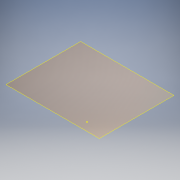
# Autodesk Inventor part: headers
Saved by Autodesk Inventor 2016 (Build 200138000, 138)
## iProperties
Created: 2016-04-08
Part Number: headers
Material: Generic
Document SubType Name: Modeling
Designer: Paschalis
Density: 1 g/cm^3
Appearance: Gold
Author: Paschalis
Autodesk Inventor part; units mm, degrees
ref_plane "YZ Plane" through (0, 0, 0) normal (1, 0, 0) x (0, 1, 0)
ref_plane "XZ Plane" through (0, 0, 0) normal (0, 1, 0) x (-1, 0, 0)
ref_plane "XY Plane" through (0, 0, 0) normal (0, 0, 1) x (1, 0, 0)
ref_plane "Work Plane1" through (-30.9119, 34.3331, -1) normal (0, 0, 1) x (-1, 0, 0)
sketch "Sketch1" plane through (-30.9119, 34.3331, -1) normal (0, 0, 1) x (-1, 0, 0)
  circle A0 centre (43.25, -35) radius 1.8 projected
  circle A1 centre (-43.25, 35) radius 1.8 projected
  circle A2 centre (-43.25, -35) radius 1.8 projected
  circle A3 centre (30.74, 18.1) radius 0.8 projected
  circle A4 centre (23.98, 18.1) radius 0.8 projected
  circle A5 centre (40.4, 18.1) radius 0.8 projected
  circle A6 centre (47.16, 18.1) radius 0.8 projected
  circle A7 centre (33.82, 25.76) radius 0.75 projected
  circle A8 centre (33.82, 35.92) radius 0.75 projected
  circle A9 centre (43.98, 25.76) radius 0.75 projected
  circle A10 centre (43.98, 35.92) radius 0.75 projected
  circle A11 centre (12.23, 25.76) radius 0.75 projected
  circle A12 centre (12.23, 35.92) radius 0.75 projected
  circle A13 centre (22.39, 25.76) radius 0.75 projected
  circle A14 centre (22.39, 35.92) radius 0.75 projected
  circle A15 centre (-36.03, -34.92) radius 0.55 projected
  circle A16 centre (-38.57, -34.92) radius 0.55 projected
  circle A17 centre (-7.7725, -36.5075) radius 0.55 projected
  circle A18 centre (40.805, -30.475) radius 0.55 projected
  circle A19 centre (-11.9, -36.19) radius 0.55 projected
  circle A20 centre (-14.44, -36.19) radius 0.55 projected
  circle A21 centre (-16.98, -36.19) radius 0.55 projected
  circle A22 centre (-11.9, -38.73) radius 0.55 projected
  circle A23 centre (-14.44, -38.73) radius 0.55 projected
  circle A24 centre (-16.98, -38.73) radius 0.55 projected
  circle A25 centre (-8.8, -11.34) radius 0.51 projected
  circle A26 centre (-11.34, -11.34) radius 0.51 projected
  circle A27 centre (-45.55, -7.62) radius 0.51 projected
  circle A28 centre (-43.01, -7.62) radius 0.51 projected
  circle A29 centre (-45.55, -10.15) radius 0.51 projected
  circle A30 centre (-43.01, -10.15) radius 0.51 projected
  circle A31 centre (-45.55, -12.7) radius 0.51 projected
  circle A32 centre (-43.01, -12.7) radius 0.51 projected
  circle A33 centre (-45.55, -15.23) radius 0.51 projected
  circle A34 centre (-43.01, -15.23) radius 0.51 projected
  circle A35 centre (-1.1, 23.5) radius 0.51 projected
  circle A36 centre (1.44, 23.5) radius 0.51 projected
  circle A37 centre (3.98, 23.5) radius 0.51 projected
  circle A38 centre (-12.22, 23.5) radius 0.51 projected
  circle A39 centre (-9.68, 23.5) radius 0.51 projected
  circle A40 centre (-7.14, 23.5) radius 0.51 projected
  circle A41 centre (3.98, 33.66) radius 0.51 projected
  circle A42 centre (1.44, 33.66) radius 0.51 projected
  circle A43 centre (-1.1, 33.66) radius 0.51 projected
  circle A44 centre (-7.14, 33.66) radius 0.51 projected
  circle A45 centre (-9.68, 33.66) radius 0.51 projected
  circle A46 centre (-12.22, 33.66) radius 0.51 projected
  circle A47 centre (-34.76, 33.03) radius 0.51 projected
  circle A48 centre (-34.76, 35.56) radius 0.51 projected
  circle A49 centre (-32.22, 33.03) radius 0.51 projected
  circle A50 centre (-32.22, 35.56) radius 0.51 projected
  circle A51 centre (-29.68, 33.03) radius 0.51 projected
  circle A52 centre (-29.68, 35.56) radius 0.51 projected
  circle A53 centre (-27.14, 33.03) radius 0.51 projected
  circle A54 centre (-27.14, 35.56) radius 0.51 projected
  circle A55 centre (-40.47, -20.31) radius 0.51 projected
  circle A56 centre (-40.47, -22.86) radius 0.51 projected
  circle A57 centre (-43.01, -20.31) radius 0.51 projected
  circle A58 centre (-43.01, -22.86) radius 0.51 projected
  circle A59 centre (-45.55, -20.31) radius 0.51 projected
  circle A60 centre (-45.55, -22.86) radius 0.51 projected
  circle A61 centre (33.82, -10.15) radius 0.51 projected
  circle A62 centre (33.82, -12.7) radius 0.51 projected
  circle A63 centre (33.82, -15.23) radius 0.51 projected
  circle A64 centre (33.82, -17.77) radius 0.51 projected
  circle A65 centre (10.33, -1.9) radius 0.51 projected
  circle A66 centre (10.33, 0.64) radius 0.51 projected
  circle A67 centre (-25.36, -29.21) radius 0.405 projected
  circle A68 centre (-30.19, -29.21) radius 0.405 projected
  circle A69 centre (19.98, -20.95) radius 0.405 projected
  circle A70 centre (24.8, -20.95) radius 0.405 projected
  circle A71 centre (40.4875, 22.5475) radius 0.3 projected
  circle A72 centre (43.98, 16.8325) radius 0.3 projected
  circle A73 centre (43.98, 19.69) radius 0.3 projected
  circle A74 centre (43.98, 22.5475) radius 0.3 projected
  circle A75 centre (47.155, 26.675) radius 0.3 projected
  circle A76 centre (47.155, 31.12) radius 0.3 projected
  circle A77 centre (43.345, 31.12) radius 0.3 projected
  circle A78 centre (47.155, 35.565) radius 0.3 projected
  circle A79 centre (47.79, 22.5475) radius 0.3 projected
  circle A80 centre (30.3275, 29.215) radius 0.3 projected
  circle A81 centre (1.435, 38.4225) radius 0.3 projected
  circle A82 centre (34.1375, 33.025) radius 0.3 projected
  circle A83 centre (21.755, 33.025) radius 0.3 projected
  circle A84 centre (25.565, 29.215) radius 0.3 projected
  circle A85 centre (21.755, 29.215) radius 0.3 projected
  circle A86 centre (25.565, 33.025) radius 0.3 projected
  circle A87 centre (30.3275, 33.025) radius 0.3 projected
  circle A88 centre (34.1375, 29.215) radius 0.3 projected
  circle A89 centre (28.105, 36.5175) radius 0.3 projected
  circle A90 centre (28.105, 25.0875) radius 0.3 projected
  circle A91 centre (-20.79, -12.3775) radius 0.3 projected
  circle A92 centre (-24.9175, -10.4725) radius 0.3 projected
  circle A93 centre (-24.6, -8.25) radius 0.3 projected
  circle A94 centre (-2.375, -13.965) radius 0.3 projected
  circle A95 centre (-30.315, -13.965) radius 0.3 projected
  circle A96 centre (-19.52, -11.425) radius 0.3 projected
  circle A97 centre (-23.33, -12.695) radius 0.3 projected
  circle A98 centre (-22.06, -6.98) radius 0.3 projected
  circle A99 centre (-12.535, -26.665) radius 0.3 projected
  circle A100 centre (-3.645, -15.235) radius 0.3 projected
  circle A101 centre (-37.3, -12.695) radius 0.3 projected
  circle A102 centre (-25.87, -12.695) radius 0.3 projected
  circle A103 centre (-36.03, -24.76) radius 0.3 projected
  circle A104 centre (-30.315, -6.98) radius 0.3 projected
  circle A105 centre (-15.075, -26.665) radius 0.3 projected
  circle A106 centre (-36.03, 1.91) radius 0.3 projected
  circle A107 centre (-34.76, -10.155) radius 0.3 projected
  circle A108 centre (-21.425, -26.03) radius 0.3 projected
  circle A109 centre (-34.76, 3.18) radius 0.3 projected
  circle A110 centre (1.435, -24.76) radius 0.3 projected
  circle A111 centre (-1.105, -19.045) radius 0.3 projected
  circle A112 centre (25.565, -17.14) radius 0.3 projected
  circle A113 centre (21.12, -17.14) radius 0.3 projected
  circle A114 centre (15.405, -6.98) radius 0.3 projected
  circle A115 centre (-5.55, -6.98) radius 0.3 projected
  circle A116 centre (-4.28, -25.395) radius 0.3 projected
  circle A117 centre (5.88, -13.965) radius 0.3 projected
  circle A118 centre (2.07, -13.965) radius 0.3 projected
  circle A119 centre (-12.535, -24.125) radius 0.3 projected
  circle A120 centre (-30.315, -15.87) radius 0.3 projected
  circle A121 centre (3.975, -8.25) radius 0.3 projected
  circle A122 centre (13.5, -8.25) radius 0.3 projected
  circle A123 centre (-33.49, -11.425) radius 0.3 projected
  circle A124 centre (-23.965, -24.125) radius 0.3 projected
  circle A125 centre (-33.49, 1.275) radius 0.3 projected
  circle A126 centre (29.375, 0.64) radius 0.3 projected
  circle A127 centre (40.805, 0.64) radius 0.3 projected
  circle A128 centre (-39.5225, -29.205) radius 0.3 projected
  circle A129 centre (-24.6, -4.44) radius 0.3 projected
  circle A130 centre (-27.775, -4.44) radius 0.3 projected
  circle A131 centre (22.39, -26.3475) radius 0.3 projected
  circle A132 centre (-13.17, 9.53) radius 0.3 projected
  circle A133 centre (-33.1725, -33.9675) radius 0.3 projected
  circle A134 centre (3.34, -26.03) radius 0.3 projected
  circle A135 centre (-14.44, -15.235) radius 0.3 projected
  circle A136 centre (-17.9325, -6.98) radius 0.3 projected
  circle A137 centre (-15.075, -3.17) radius 0.3 projected
  circle A138 centre (-46.825, 8.26) radius 0.3 projected
  circle A139 centre (0.8, -11.1075) radius 0.3 projected
  circle A140 centre (-9.36, -16.505) radius 0.3 projected
  circle A141 centre (12.865, -19.045) radius 0.3 projected
  circle A142 centre (38.9, -24.76) radius 0.3 projected
  circle A143 centre (42.075, -10.79) radius 0.3 projected
  circle A144 centre (34.455, 9.53) radius 0.3 projected
  circle A145 centre (38.9, -6.345) radius 0.3 projected
  circle A146 centre (-28.41, 28.58) radius 0.3 projected
  circle A147 centre (-22.06, 28.58) radius 0.3 projected
  circle A148 centre (-47.46, 17.4675) radius 0.3 projected
  circle A149 centre (27.47, 18.1025) radius 0.3 projected
  circle A150 centre (32.2325, 20.96) radius 0.3 projected
  circle A151 centre (27.47, 15.88) radius 0.3 projected
  circle A152 centre (27.47, 20.325) radius 0.3 projected
  circle A153 centre (22.39, 20.96) radius 0.3 projected
  circle A154 centre (21.4375, 18.42) radius 0.3 projected
  circle A155 centre (-2.375, 13.34) radius 0.3 projected
  circle A156 centre (11.9125, 31.12) radius 0.3 projected
  circle A157 centre (12.23, 20.325) radius 0.3 projected
  circle A158 centre (14.77, 23.5) radius 0.3 projected
  circle A159 centre (9.69, 23.5) radius 0.3 projected
  circle A160 centre (14.135, 29.215) radius 0.3 projected
  circle A161 centre (9.69, 29.215) radius 0.3 projected
  circle A162 centre (14.135, 32.7075) radius 0.3 projected
  circle A163 centre (9.69, 32.7075) radius 0.3 projected
  circle A164 centre (7.785, 15.88) radius 0.3 projected
  circle A165 centre (14.77, -9.52) radius 0.3 projected
  circle A166 centre (-22.06, -11.425) radius 0.3 projected
  circle A167 centre (-0.47, -5.075) radius 0.3 projected
  circle A168 centre (-0.47, -12.06) radius 0.3 projected
  circle A169 centre (-40.1575, 2.8625) radius 0.3 projected
  circle A170 centre (-32.22, 9.53) radius 0.3 projected
  circle A171 centre (-6.82, -5.075) radius 0.3 projected
  circle A172 centre (45.885, -16.505) radius 0.3 projected
  circle A173 centre (41.44, -16.505) radius 0.3 projected
  circle A174 centre (36.995, -8.885) radius 0.3 projected
  circle A175 centre (45.25, -8.885) radius 0.3 projected
  circle A176 centre (-43.65, 0.9575) radius 0.3 projected
  circle A177 centre (-20.155, -5.075) radius 0.3 projected
  circle A178 centre (-26.1875, -6.345) radius 0.3 projected
  circle A179 centre (-23.965, 31.12) radius 0.3 projected
  circle A180 centre (-32.22, 14.61) radius 0.3 projected
  circle A181 centre (-39.84, 22.23) radius 0.3 projected
  circle A182 centre (-43.65, 23.5) radius 0.3 projected
  circle A183 centre (9.69, -13.965) radius 0.3 projected
  circle A184 centre (44.2975, -27.935) radius 0.3 projected
  circle A185 centre (-27.14, -19.045) radius 0.3 projected
  circle A186 centre (-30.315, -22.22) radius 0.3 projected
  line L0 (-50, -40) -> (50, -40) projected
  line L1 (50, -40) -> (50, 40) projected
  line L2 (50, 40) -> (-50, 40) projected
  line L3 (-50, 40) -> (-50, -40) projected
  point P0 (-30.9119, 34.3331)
extrude "Extrusion1" add sketch "Sketch1" along normal blind 8 contours A25 | A26 | A27 | A28 | A29 | A30 | A31 | A32 | A33 | A34 | A47 | A48 | A49 | A50 | A51 | A52 | A53 | A54 | A55 | A56 | A57 | A58 | A59 | A60
body "Solid1"
